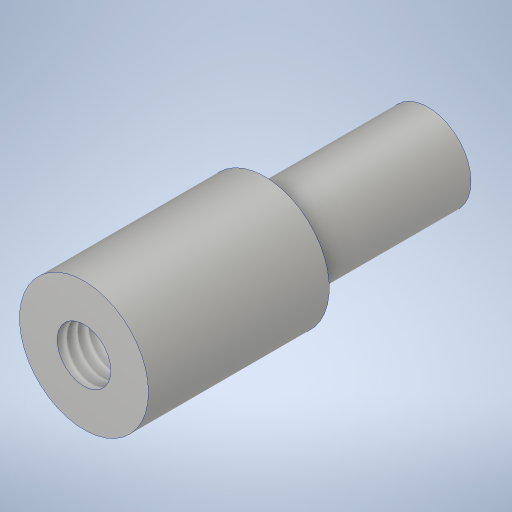
# Autodesk Inventor part: EL2-008
Saved by Autodesk Inventor 2023.4 (Build 274418000, 418)
## iProperties
Created: 2025-01-11
Part Number: EL2-008
Material: Aluminum 6061
Document SubType Name: Modeling
Designer: mavericks
Density: 2.7 g/cm^3
Appearance: Aluminum - Flat
Author: mavericks
Autodesk Inventor part; units mm, degrees
ref_plane "YZ Plane" through (0, 0, 0) normal (1, 0, 0) x (0, 1, 0)
ref_plane "XZ Plane" through (0, 0, 0) normal (0, 1, 0) x (-1, 0, 0)
ref_plane "XY Plane" through (0, 0, 0) normal (0, 0, 1) x (1, 0, 0)
sketch "Sketch1" plane through (0, 0, 0) normal (0, 0, 1) x (1, 0, 0)
  circle A0 centre (0, 0) radius 4.7625
  dimension "d0" = 9.525
  constraints: 1 centre point, 1 coincident
  measures "d0" diameter of A0
extrude "Extrusion1" add sketch "Sketch1" along normal mid plane 25.4
sketch "Sketch3" plane through (0, 0, 12.7) normal (0, 0, 1) x (1, 0, 0)
  circle A0 centre (0, 0) radius 4.7625 projected
  constraints: 1 coincident
hole "Hole1" at (0, 0, 12.7) direction (0, 0, -1) diameter 3.9624 depth 13.6144 tip angle 118 thread size "10-32 UNF" class "2B" standard "ANSI Unified Screw Threads"
sketch "Sketch4" plane through (0, 0, -12.7) normal (0, 0, -1) x (-1, 0, 0)
  circle A0 centre (0, 0) radius 3.175
  circle A1 centre (0, 0) radius 4.7625 projected
  dimension "d10" = 6.35
  constraints: 1 centre point, 1 coincident
  measures "d10" diameter of A0
extrude "Extrusion2" cut sketch "Sketch4" against normal blind 12.0523
body "Solid1"
